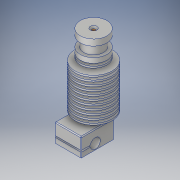
# Autodesk Inventor part: e3dv6
Saved by Autodesk Inventor 2017 (Build 210142000, 142)
## iProperties
Created: 2016-04-03
Part Number: e3dv6
Material: Generic
Document SubType Name: Modeling
Designer: brent
Density: 1 g/cm^3
Appearance: Aluminum - Flat
Author: brent
Autodesk Inventor part; units mm, degrees
ref_plane "YZ Plane" through (0, 0, 0) normal (1, 0, 0) x (0, 1, 0)
ref_plane "XZ Plane" through (0, 0, 0) normal (0, 1, 0) x (-1, 0, 0)
ref_plane "XY Plane" through (0, 0, 0) normal (0, 0, 1) x (1, 0, 0)
sketch "Sketch2" plane through (0, 0, 0) normal (0, 0, 1) x (1, 0, 0)
  line L0 (0, 0) -> (0, -42.7)
  line L1 (0, 0) -> (-8, 0)
  line L2 (-8, 0) -> (-8, -3.7)
  line L3 (-8, -3.7) -> (0, -3.7)
  line L4 (0, -3.7) -> (0, 0)
  line L5 (0, -3.7) -> (-6, -3.7)
  line L6 (-6, -3.7) -> (-6, -9.7)
  line L7 (-6, -9.7) -> (0, -9.7)
  line L8 (0, -9.7) -> (0, -3.7)
  line L9 (0, -9.7) -> (-8, -9.7)
  line L10 (-8, -9.7) -> (-8, -12.7)
  line L11 (-8, -12.7) -> (0, -12.7)
  line L12 (0, -12.7) -> (0, -9.7)
  line L13 (0, -42.7) -> (-11.15, -42.7)
  line L14 (-11.15, -42.7) -> (-11.15, -41.7)
  line L15 (-11.15, -41.7) -> (0, -41.7)
  line L16 (0, -41.7) -> (0, -42.7)
  line L17 (-11.15, -39.2) -> (0, -39.2)
  line L18 (0, -39.2) -> (0, -40.2)
  line L19 (0, -40.2) -> (-11.15, -40.2)
  line L20 (-11.15, -40.2) -> (-11.15, -39.2)
  line L21 (-11.15, -36.7) -> (0, -36.7)
  line L22 (0, -36.7) -> (0, -37.7)
  line L23 (0, -37.7) -> (-11.15, -37.7)
  line L24 (-11.15, -37.7) -> (-11.15, -36.7)
  line L25 (-11.15, -34.2) -> (0, -34.2)
  line L26 (0, -34.2) -> (0, -35.2)
  line L27 (0, -35.2) -> (-11.15, -35.2)
  line L28 (-11.15, -35.2) -> (-11.15, -34.2)
  line L29 (-11.15, -31.7) -> (0, -31.7)
  line L30 (0, -31.7) -> (0, -32.7)
  line L31 (0, -32.7) -> (-11.15, -32.7)
  line L32 (-11.15, -32.7) -> (-11.15, -31.7)
  line L33 (-11.15, -29.2) -> (0, -29.2)
  line L34 (0, -29.2) -> (0, -30.2)
  line L35 (0, -30.2) -> (-11.15, -30.2)
  line L36 (-11.15, -30.2) -> (-11.15, -29.2)
  line L37 (-11.15, -26.7) -> (0, -26.7)
  line L38 (0, -26.7) -> (0, -27.7)
  line L39 (0, -27.7) -> (-11.15, -27.7)
  line L40 (-11.15, -27.7) -> (-11.15, -26.7)
  line L41 (-11.15, -24.2) -> (0, -24.2)
  line L42 (0, -24.2) -> (0, -25.2)
  line L43 (0, -25.2) -> (-11.15, -25.2)
  line L44 (-11.15, -25.2) -> (-11.15, -24.2)
  line L45 (-11.15, -21.7) -> (0, -21.7)
  line L46 (0, -21.7) -> (0, -22.7)
  line L47 (0, -22.7) -> (-11.15, -22.7)
  line L48 (-11.15, -22.7) -> (-11.15, -21.7)
  line L49 (-11.15, -19.2) -> (0, -19.2)
  line L50 (0, -19.2) -> (0, -20.2)
  line L51 (0, -20.2) -> (-11.15, -20.2)
  line L52 (-11.15, -20.2) -> (-11.15, -19.2)
  line L53 (-11.15, -16.7) -> (0, -16.7)
  line L54 (0, -16.7) -> (0, -17.7)
  line L55 (0, -17.7) -> (-11.15, -17.7)
  line L56 (-11.15, -17.7) -> (-11.15, -16.7)
  line L57 (0, -14.2) -> (-8, -14.2)
  line L58 (-8, -14.2) -> (-8, -15.2)
  line L59 (-8, -15.2) -> (0, -15.2)
  line L60 (0, -15.2) -> (0, -14.2)
  line L61 (0, -12.7) -> (0, -39.2)
  line L62 (-4, -15.2) -> (-4, -16.7)
  line L63 (-4, -14.2) -> (-4, -12.7)
  line L64 (-4, -16.7) -> (-6, -41.7)
  line L65 (-4.2, -17.7) -> (-4.2, -19.2)
  line L66 (-4.4, -21.7) -> (-4.4, -20.2)
  line L67 (-4.6, -24.2) -> (-4.6, -22.7)
  line L68 (-4.8, -26.7) -> (-4.8, -25.2)
  line L69 (-5, -29.2) -> (-5, -27.7)
  line L70 (-5.2, -31.7) -> (-5.2, -30.2)
  line L71 (-5.4, -34.2) -> (-5.4, -32.7)
  line L72 (-5.6, -36.7) -> (-5.6, -35.2)
  line L73 (-5.8, -39.2) -> (-5.8, -37.7)
  line L74 (-6, -41.7) -> (-6, -40.2)
  line L75 (0, -17.7) -> (0, -41.7)
  line L76 (0, -12.7) -> (0, -14.2)
  line L77 (0, -15.2) -> (0, -16.7)
  line L78 (0, -30.2) -> (0, -31.7)
  line L79 (0, -42.7) -> (-2, -42.7)
  line L80 (-2, -42.7) -> (-2, -49.8)
  line L81 (-2, -49.8) -> (0, -49.8)
  line L82 (0, -49.8) -> (0, -42.7)
  line L83 (0, -49.8) -> (-3, -49.8)
  line L84 (-3, -49.8) -> (-3, -55.8)
  line L85 (-3, -55.8) -> (0, -55.8)
  line L86 (0, -55.8) -> (0, -49.8)
  line L87 (0, -55.8) -> (-2.5, -55.8)
  line L88 (-2.5, -55.8) -> (-2.5, -57.3)
  line L89 (-2.5, -57.3) -> (0, -57.3)
  line L90 (0, -57.3) -> (0, -55.8)
  line L91 (0, -57.3) -> (-3.5, -57.3)
  line L92 (-3.5, -57.3) -> (-3.5, -60.3)
  line L93 (-3.5, -60.3) -> (0, -60.3)
  line L94 (0, -60.3) -> (0, -57.3)
  line L95 (-1.9004, -60.3) -> (-0.5, -62.3)
  line L96 (-0.5, -62.3) -> (0, -62.3)
  line L97 (0, -62.3) -> (0, -60.3)
  dimension "d21" = 42.7
  dimension "d22" = 8
  dimension "d23" = 3.7
  dimension "d24" = 6
  dimension "d25" = 6
  dimension "d26" = 8
  dimension "d27" = 3
  dimension "d28" = 11.15
  dimension "d29" = 1
  dimension "d39" = 2.5
  dimension "d44" = 8
  dimension "d45" = 1
  dimension "d46" = 1.5
  dimension "d48" = 12
  dimension "d50" = 2
  dimension "d51" = 7.1
  dimension "d52" = 3
  dimension "d53" = 6
  dimension "d54" = 2.5
  dimension "d55" = 1.5
  dimension "d56" = 3.5
  dimension "d57" = 10.5
  dimension "d58" = 125
  dimension "d59" = 0.5
  dimension "d60" = 2
  constraints: 194 end point, 22 equal length, 22 point on line, 17 perpendicular, 10 horizontal, 7 vertical, 3 midpoint, 92 other
  measures "d21" distance of L0.start L0.end
  measures "d22" distance of L3.end L2.end
  measures "d23" distance of L2.end L1.end
  measures "d24" distance of L7.end L6.end
  measures "d25" distance of L6.end L5.end
  measures "d26" distance of L11.end L10.end
  measures "d27" distance of L10.end L9.end
  measures "d28" distance of L14.end L15.end
  measures "d29" distance of L13.end L14.end
  measures "d39" distance of L15.end L17.end
  measures "d44" distance of L59.end L58.end
  measures "d45" distance of L58.end L57.end
  measures "d46" distance between parallel lines of L11 L57
  measures "d48" diameter of L74.start L0
  measures "d50" distance of L81.end L80.end
  measures "d51" distance of L80.end L79.end
  measures "d52" distance of L85.end L84.end
  measures "d53" distance of L84.end L83.end
  measures "d54" distance of L89.end L88.end
  measures "d55" distance of L88.end L87.end
  measures "d56" distance of L93.end L92.end
  measures "d57" distance between parallel lines of L83 L93
  measures "d58" angle of L93 L95
  measures "d59" distance of L95.end L96.end
  measures "d60" distance of L96.end L93.end
revolve "Revolution1" add sketch "Sketch2" angle 360 about axis through (0, -31.7, 0) along (0, -1, 0)
sketch "Sketch3" plane through (0, -60.3, 0) normal (0, -1, 0) x (1, 0, 0)
  circle A0 centre (0, 0) radius 3.5 projected
  circle A1 centre (0, 0) radius 1.9004 projected
  line L0 (4.0415, 0) -> (2.0207, -3.5)
  line L1 (2.0207, -3.5) -> (-2.0207, -3.5)
  line L2 (-2.0207, -3.5) -> (-4.0415, 0)
  line L3 (-4.0415, 0) -> (-2.0207, 3.5)
  line L4 (-2.0207, 3.5) -> (2.0207, 3.5)
  line L5 (2.0207, 3.5) -> (4.0415, 0)
  circle A2 centre (0, 0) radius 12.5
  dimension "d61" = 7
  dimension "d62" = 25
  constraints: 12 end point, 2 coincident, 1 centre point, 1 horizontal, 13 other
  measures "d61" distance between parallel lines of L1 L4
  measures "d62" diameter of A2
extrude "Extrusion1" add sketch "Sketch3" against normal up to surface (3 mm away) contours A0 L5 L0 | A0 L4 L5 | L0 L1 A0 | A0 L3 L4 | L1 L2 A0 | A0 L2 L3
sketch "Sketch4" plane through (0, 0, 0) normal (1, 0, 0) x (0, 1, 0)
  line L0 (-45.05, 15.5) -> (-56.55, 15.5)
  line L1 (-56.55, 15.5) -> (-56.55, -4.5)
  line L2 (-56.55, -4.5) -> (-45.05, -4.5)
  line L3 (-45.05, -4.5) -> (-45.05, 15.5)
  arc A0 (-53.05, 9.9834) -> (-52.05, 9.9834) centre (-52.55, 7) ccw
  line L4 (-60.3, 0) -> (-57.3, 0) projected
  line L5 (-52.55, 7) -> (-52.55, 15.5) construction
  line L6 (-53.05, 15.5) -> (-53.05, 9.9834)
  line L7 (-52.05, 9.9834) -> (-52.05, 15.5)
  line L8 (-57.3, 2.5) -> (-55.8, 2.5) projected
  point P0 (0, 0)
  point P1 (-52.55, 11.25)
  point P2 (-56.55, 2.5)
  dimension "d65" = 11.5
  dimension "d66" = 20
  dimension "d67" = 6.05
  dimension "d68" = 4
  dimension "d69" = 11.5
  dimension "d70" = 4.5
  dimension "d84" = 3.5
  dimension "d85" = 4.5
  constraints: 16 end point, 4 parallel, 4 point on line, 2 midpoint, 2 perpendicular, 2 point on circle, 1 centre point, 1 horizontal
  measures "d65" distance of L2.end L1.end
  measures "d66" distance of L1.end L0.end
  measures "d67" diameter of A0
  measures "d68" distance from line of L1 L5.start
  measures "d69" distance from line of L2 L5.start
  measures "d70" distance between parallel lines of L4 L2
  measures "d84" distance between parallel lines of L1 L6
  measures "d85" distance between parallel lines of L1 L7
extrude "Extrusion2" add sketch "Sketch4" along normal mid plane 16 contours L3 L2 L1 L0 L6 A0 L7
sketch "Sketch5" plane through (0, -62.3, 0) normal (0, -1, 0) x (1, 0, 0)
  circle A0 centre (0, 0) radius 0.2
  dimension "d75" = 0.4
  constraints: 1 centre point, 1 coincident
  measures "d75" diameter of A0
extrude "Extrusion3" cut sketch "Sketch5" against normal through all
sketch "Sketch6" plane through (0, 0, 0) normal (0, 1, 0) x (1, 0, 0)
  circle A0 centre (0, 0) radius 1
  dimension "d78" = 2
  constraints: 1 centre point, 1 coincident
  measures "d78" diameter of A0
extrude "Extrusion4" cut sketch "Sketch6" against normal up to surface (60.3 mm away)
chamfer "Chamfer1" distance 1 angle 45 1 edges at (-1, 0, 0)
chamfer "Chamfer2" distance 0.5 angle 45 14 edges at (-8, -56.55, 5.5) (0, -56.55, 15.5) (-8, -54.8, 15.5) (-8, -48.55, 15.5) (8, -48.55, 15.5) (0, -45.05, 15.5) (-8, -45.05, 5.5) (-8, -50.8, -4.5) (0, -56.55, -4.5) (8, -56.55, 5.5) (8, -50.8, -4.5) (8, -45.05, 5.5) (8, -54.8, 15.5) (0, -45.05, -4.5)
sketch "Sketch7" plane through (0, 0, 0) normal (0, 0, 1) x (1, 0, 0)
  line L0 (-4.0415, -60.3) -> (-2.0207, -60.3) projected
  line L1 (-4.0415, -60.3) -> (-4.0415, -57.3) projected
  line L2 (-4.0415, -60.05) -> (-3.7915, -60.3)
  line L3 (0, -74.76) -> (0, 12.46) projected
  line L4 (-2.0207, -57.3) -> (-4.0415, -57.3) projected
  line L5 (-4.0415, -57.55) -> (-3.7915, -57.3)
  point P0 (0, 0)
  dimension "d89" = 0.25
  dimension "d90" = 0.25
  dimension "d92" = 0.25
  dimension "d93" = 0.25
  constraints: 4 end point, 4 point on line
  measures "d89" distance from line of L0 L2.start
  measures "d90" distance from line of L1 L2.end
  measures "d92" distance of L1.end L5.start
  measures "d93" distance of L5.end L1.end
revolve "Revolution2" cut sketch "Sketch7" angle 360 about axis through (0, -10, 0) along (0, 1, 0)
equation "\"d90\" = d89"
equation "\"d92\" = d89"
equation "\"d93\" = d89"
body "Solid1"
